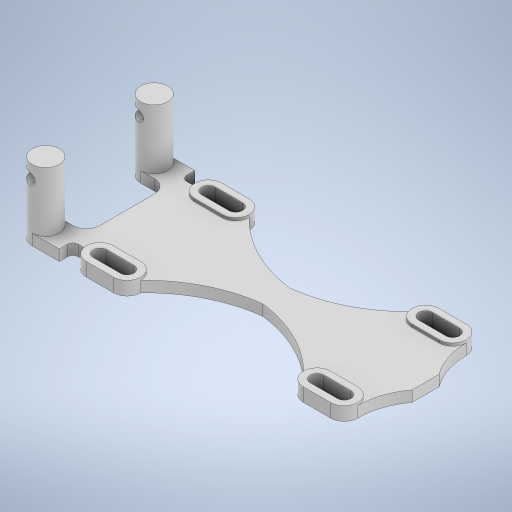
# Autodesk Inventor part: WPNB
Saved by Autodesk Inventor 2024 (Build 280153000, 153)
## iProperties
Created: 2025-10-03
Part Number: WPNB
Material: Generic
Document SubType Name: Modeling
Designer: albah
Density: 1 g/cm^3
Appearance: Default
Author: albah
Autodesk Inventor part; units mm, degrees
ref_plane "YZ Plane" through (0, 0, 0) normal (1, 0, 0) x (0, 1, 0)
ref_plane "XZ Plane" through (0, 0, 0) normal (0, 1, 0) x (-1, 0, 0)
ref_plane "XY Plane" through (0, 0, 0) normal (0, 0, 1) x (1, 0, 0)
sketch "Sketch1" plane through (0, 0, 0) normal (0, 1, 0) x (-1, 0, 0)
  line L0 (75, 5) -> (75, -5)
  line L1 (75, -5) -> (20, -5)
  line L2 (-75, 5) -> (75, -5) construction
  line L3 (75, 5) -> (-75, -5) construction
  line L4 (65, -20) -> (55, -20) construction
  line L5 (65, -17.5) -> (55, -17.5)
  line L6 (55, -22.5) -> (65, -22.5)
  arc A0 (65, -22.5) -> (65, -17.5) centre (65, -20) ccw
  arc A1 (55, -17.5) -> (55, -22.5) centre (55, -20) ccw
  line L7 (65, 20) -> (55, 20) construction
  line L8 (65, 22.5) -> (55, 22.5)
  line L9 (55, 17.5) -> (65, 17.5)
  arc A2 (65, 17.5) -> (65, 22.5) centre (65, 20) ccw
  arc A3 (55, 22.5) -> (55, 17.5) centre (55, 20) ccw
  line L10 (65, -20) -> (55, -20) construction
  line L11 (65, -15) -> (55, -15)
  line L12 (55, -25) -> (65, -25)
  arc A4 (65, -25) -> (65, -15) centre (65, -20) ccw
  arc A5 (55, -15) -> (55, -25) centre (55, -20) ccw
  line L13 (65, 20) -> (55, 20) construction
  line L14 (65, 25) -> (55, 25)
  line L15 (55, 15) -> (65, 15)
  arc A6 (65, 15) -> (65, 25) centre (65, 20) ccw
  arc A7 (55, 25) -> (55, 15) centre (55, 20) ccw
  arc A8 (70, 20) -> (75, 5) centre (95, 20) ccw
  arc A9 (75, -5) -> (70, -20) centre (95, -20) ccw
  line L16 (20, 0) -> (20, -5)
  arc A10 (50, -20) -> (20, -5) centre (13.9346, -54.6307) ccw
  arc A11 (20, 5) -> (50, 20) centre (13.9346, 54.6307) ccw
  line L17 (20, 5) -> (75, 5)
  line L18 (7.8693, 5) -> (20, 5)
  line L19 (-25, 17.5) -> (-15, 17.5)
  line L20 (-25, 20) -> (-15, 20) construction
  line L21 (-15, 22.5) -> (-25, 22.5)
  arc A12 (-15, 15) -> (-15, 25) centre (-15, 20) ccw
  arc A13 (-15, 17.5) -> (-15, 22.5) centre (-15, 20) ccw
  arc A14 (-30, -20) -> (-35, -5) centre (-55, -20) ccw
  arc A15 (-25, 22.5) -> (-25, 17.5) centre (-25, 20) ccw
  line L22 (-25, -20) -> (-15, -20) construction
  line L23 (-15, -17.5) -> (-25, -17.5)
  line L24 (-15, -15) -> (-25, -15)
  line L25 (-25, -20) -> (-15, -20) construction
  line L26 (-25, -22.5) -> (-15, -22.5)
  arc A16 (-25, -17.5) -> (-25, -22.5) centre (-25, -20) ccw
  arc A17 (-15, -22.5) -> (-15, -17.5) centre (-15, -20) ccw
  arc A18 (-15, -25) -> (-15, -15) centre (-15, -20) ccw
  line L27 (-25, -25) -> (-15, -25)
  arc A19 (-25, -15) -> (-25, -25) centre (-25, -20) ccw
  line L28 (-35, -5) -> (-35, 5)
  arc A20 (-10, 20) -> (20, 5) centre (26.0654, 54.6307) ccw
  line L29 (-35, 5) -> (20, 5)
  arc A21 (20, -5) -> (-10, -20) centre (26.0654, -54.6307) ccw
  line L30 (20, -5) -> (-35, -5)
  line L31 (-25, 15) -> (-15, 15)
  line L32 (-25, 20) -> (-15, 20) construction
  line L33 (-15, 25) -> (-25, 25)
  arc A22 (-35, 5) -> (-30, 20) centre (-55, 20) ccw
  arc A23 (-25, 25) -> (-25, 15) centre (-25, 20) ccw
  line L34 (115, -5) -> (-35, 5) construction
  line L35 (-35, -5) -> (115, 5) construction
  line L36 (75, 0) -> (75, -20)
  line L37 (75, 0) -> (75, 20)
  line L38 (75, 20) -> (90, 20)
  line L39 (90, 20) -> (90, 15)
  line L40 (90, 15) -> (75, 15)
  line L41 (75, 15) -> (75, 20)
  line L42 (75, 20) -> (90, 20)
  line L43 (90, 20) -> (90, 25)
  line L44 (90, 25) -> (75, 25)
  line L45 (75, 25) -> (75, 22)
  line L46 (75, -20) -> (90, -20)
  line L47 (90, -20) -> (90, -15)
  line L48 (90, -15) -> (75, -15)
  line L49 (75, -15) -> (75, -20)
  line L50 (75, -20) -> (90, -20)
  line L51 (90, -20) -> (90, -25)
  line L52 (90, -25) -> (75, -25)
  line L53 (75, -25) -> (75, -22)
  line L54 (73, -20) -> (70, -20)
  arc A24 (75, -22) -> (73, -20) centre (73, -22) ccw
  line L55 (73, 20) -> (70, 20)
  arc A25 (73, 20) -> (75, 22) centre (73, 22) ccw
  point P0 (0, 0)
  point P1 (60, -20)
  point P2 (60, 20)
  point P3 (60, -20)
  point P4 (60, 20)
  point P5 (0, 0)
  point P6 (-20, 20)
  point P7 (-20, -20)
  point P8 (-20, -20)
  point P9 (-35, 0)
  point P10 (32.1307, -5)
  point P11 (-20, 20)
  point P12 (40, 0)
  point P13 (20, 5)
  dimension "d1" = 10
  dimension "d16" = 10
  dimension "d17" = 5
  dimension "d18" = 5
  dimension "d20" = 10
  dimension "d21" = 10
  dimension "d22" = 25
  dimension "d23" = 25
  dimension "d26" = 50
  dimension "d28" = 50
  dimension "d32" = 360
  dimension "d34" = 55
  dimension "d35" = 42.5
  dimension "d36" = 25
  dimension "d37" = 42.8693
  dimension "d38" = 55
  dimension "d39" = 55
  dimension "d40" = 86.186
  dimension "d41" = 86.186
  dimension "d42" = 40
  dimension "d43" = 40
  dimension "d44" = 55
  dimension "d45" = 5
  dimension "d46" = 45
  dimension "d47" = 15
  dimension "d48" = 5
  dimension "d49" = 0
  dimension "d50" = 2
  dimension "d51" = 2
  constraints: 128 end point, 59 point on circle, 28 tangent, 26 centre point, 15 parallel, 8 midpoint, 8 perpendicular, 6 point on line, 4 collinear, 4 horizontal, 3 coincident, 2 vertical, 145 other
  measures "d1" distance of L0.start L0.end
  measures "d16" distance of L4.start L4.end
  measures "d17" diameter of A1
  measures "d18" diameter of A3
  measures "d20" diameter of A5
  measures "d21" diameter of A7
  measures "d22" radius of A8
  measures "d23" radius of A9
  measures "d26" radius of A10
  measures "d28" radius of A11
  measures "d34" distance between parallel lines of L0 L16
  measures "d35" distance between parallel lines of L14 L5
  measures "d36" distance from line of A10.start L0
  measures "d37" distance from line of point (32.131, -5) L0
  measures "d38" distance from line of L17.start L0
  measures "d39" distance from line of L29.end L0
  measures "d40" angle of L35 L0
  measures "d41" angle of L34 L0
  measures "d42" distance from line of L35.end L0
  measures "d43" distance from line of L34.start L0
  measures "d44" distance from line of A11.start L0
  measures "d45" distance from line of L37.end L14
  measures "d46" distance from line of L36.end L14
  measures "d47" distance of L37.end L38.end
  measures "d48" distance of L38.end L39.end
  measures "d49" distance between parallel lines of L51 L39
  measures "d50" radius of A24
  measures "d51" radius of A25
extrude "Extrusion1" add sketch "Sketch1" along normal blind 4 contours L17 A11 A7 L15 A6 A8 | L0 L1 L30 L28 L29 L18 L17 | A8 L55 A25 L45 L44 L43 L38 L37 | L18 L29 A22 A23 L31 A12 A20 | L37 L38 L39 L40 | A9 A4 L11 A5 A10 L1 | L36 L46 L51 L52 L53 A24 L54 A9 | A21 A18 L24 A19 A14 L30 | L48 L47 L46 L36
extrude "Extrusion2" add sketch "Sketch1" along normal blind 5 contours A6 L15 A7 L14 | A12 L31 A23 L33 | A4 L12 A5 L11 | A18 L27 A19 L24
fillet "Fillet1" radius 5 2 edges at (-75, 2, -15) (-75, 2, 15)
sketch "Sketch2" plane through (0, 4, 0) normal (0, 1, 0) x (1, 0, 0)
  line L0 (-80, -15) -> (-90, -15) projected
  line L1 (-90, -25) -> (-75, -25) projected
  line L2 (-90, -15) -> (-90, -25)
  line L3 (-90, -25) -> (-80, -25)
  line L4 (-80, -25) -> (-80, -15)
  line L5 (-80, -15) -> (-90, -15)
  line L6 (-90, 15) -> (-80, 15) projected
  line L7 (-75, 25) -> (-90, 25) projected
  line L8 (-90, 15) -> (-90, 25)
  line L9 (-90, 25) -> (-80, 25)
  line L10 (-80, 25) -> (-80, 15)
  line L11 (-80, 15) -> (-90, 15)
  point P0 (0, 0)
  dimension "d57" = 10
  dimension "d58" = 0
  constraints: 16 end point, 4 parallel, 4 perpendicular
  measures "d57" distance of L3.end L1.start
  measures "d58" distance between parallel lines of L10 L4
extrude "Extrusion3" add sketch "Sketch2" along normal blind 22
sketch "Sketch3" plane through (-90, 0, 25) normal (0, 0, 1) x (1, 0, 0)
  line L0 (0, 0) -> (0, 26) projected
  line L1 (0, 21) -> (4, 21) construction
  line L2 (0, 19) -> (4, 19)
  line L3 (4, 23) -> (0, 23)
  arc A0 (0, 23) -> (0, 19) centre (0, 21) ccw
  arc A1 (4, 19) -> (4, 23) centre (4, 21) ccw
  point P0 (90, 0)
  point P1 (2, 21)
  dimension "d61" = 5
  dimension "d62" = 4
  dimension "d63" = 4
  constraints: 8 end point, 4 point on circle, 4 tangent, 2 centre point, 1 midpoint, 1 parallel, 1 perpendicular, 1 point on line
  measures "d61" distance of L0.end L1.start
  measures "d62" distance of L1.start L1.end
  measures "d63" diameter of A1
extrude "Extrusion4" cut sketch "Sketch3" against normal through all
fillet "Fillet2" radius 5 12 edges at (-90, 9.5, 25) (-90, 9.5, 15) (-90, 24.5, 25) (-90, 24.5, 15) (-90, 9.5, -15) (-90, 9.5, -25) (-90, 24.5, -15) (-90, 24.5, -25) (-80, 15, -15) (-80, 15, -25) (-80, 15, 15) (-80, 15, 25)
body "Solid1"
